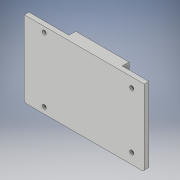
# Autodesk Inventor part: BeagleBoneMountingBracket
Saved by Autodesk Inventor 2019.3 (Build 233278000, 278)
## iProperties
Created: 2019-02-16
Part Number: BeagleBoneMountingBracket
Material: Generic
Document SubType Name: Modeling
Designer: mark
Density: 1 g/cm^3
Appearance: Default
Author: mark
Autodesk Inventor part; units mm, degrees
ref_plane "YZ Plane" through (0, 0, 0) normal (1, 0, 0) x (0, 1, 0)
ref_plane "XZ Plane" through (0, 0, 0) normal (0, 1, 0) x (-1, 0, 0)
ref_plane "XY Plane" through (0, 0, 0) normal (0, 0, 1) x (1, 0, 0)
sketch "Sketch1" plane through (0, 0, 0) normal (0, 0, 1) x (1, 0, 0)
  line L0 (0, 0) -> (90, 0)
  line L1 (90, 0) -> (90, 57)
  line L2 (90, 57) -> (0, 57)
  line L3 (0, 57) -> (0, 0)
  circle A0 centre (15, 53) radius 1.55
  circle A1 centre (15, 4.74) radius 1.55
  circle A2 centre (80.699, 49.825) radius 1.55
  circle A3 centre (80.699, 7.915) radius 1.55
  dimension "d0" = 57
  dimension "d1" = 90
  dimension "d2" = 3.1
  dimension "d3" = 3.1
  dimension "d4" = 3.1
  dimension "d5" = 3.1
  dimension "d6" = 4
  dimension "d7" = 15
  dimension "d8" = 48.26
  dimension "d9" = 15
  dimension "d10" = 80.699
  dimension "d11" = 7.175
  dimension "d12" = 41.91
  dimension "d13" = 80.699
  constraints: 8 end point, 4 centre point, 2 horizontal, 2 vertical
  measures "d0" distance between parallel lines of L0 L2
  measures "d1" distance between parallel lines of L1 L3
  measures "d2" diameter of A0
  measures "d3" diameter of A1
  measures "d4" diameter of A2
  measures "d5" diameter of A3
  measures "d6" distance from line of L2 A0.centre
  measures "d7" distance from line of A0.centre L3
  measures "d8" distance of A1.centre A0.centre
  measures "d9" distance from line of A1.centre L3
  measures "d10" distance from line of L3 A2.centre
  measures "d11" distance from line of L2 A2.centre
  measures "d12" distance of A3.centre A2.centre
  measures "d13" distance from line of A3.centre L3
extrude "Extrusion1" add sketch "Sketch1" along normal blind 3.5
sketch "Sketch2" plane through (0, 0, 0) normal (0, 0, -1) x (-1, 0, 0)
  line L0 (-70, 35) -> (-30, 35)
  line L1 (-30, 35) -> (-30, 57)
  line L2 (-30, 57) -> (-70, 57)
  line L3 (-70, 57) -> (-70, 35)
  line L4 (0, 0) -> (-90, 0) projected
  line L5 (-90, 57) -> (0, 57) projected
  line L6 (-90, 0) -> (-90, 57) projected
  dimension "d16" = 35
  dimension "d17" = 40
  dimension "d18" = 20
  constraints: 8 end point, 2 horizontal, 2 vertical, 1 collinear
  measures "d16" distance between parallel lines of L0 L4
  measures "d17" distance between parallel lines of L1 L3
  measures "d18" distance between parallel lines of L6 L3
extrude "Extrusion2" add sketch "Sketch2" along normal blind 5.1
sketch "Sketch3" plane through (30, 35, 0) normal (0, -1, 0) x (1, 0, 0)
  line L0 (0, -5.1) -> (40, -5.1)
  line L1 (40, -5.1) -> (40, -3.1)
  line L2 (40, -3.1) -> (0, -3.1)
  line L3 (0, -3.1) -> (0, -5.1)
  line L4 (40, -5.1) -> (0, -5.1) projected
  line L5 (0, 0) -> (0, -5.1) projected
  line L6 (40, 0) -> (40, -5.1) projected
  line L7 (-30, 0) -> (60, 0) projected
  dimension "d21" = 3.1
  constraints: 8 end point, 3 collinear
  measures "d21" distance between parallel lines of L7 L2
extrude "Extrusion3" add sketch "Sketch3" along normal blind 25 contours L3 L2 L1 L0
chamfer "Chamfer1" distance 5 angle 45 2 edges at (70, 10, -4.1) (30, 10, -4.1)
chamfer "Chamfer2" distance 1 angle 45 2 edges at (90, 0, 1.75) (0, 0, 1.75)
chamfer "Chamfer3" distance 2 angle 45 4 edges at (13.45, 53, 0) (13.45, 4.74, 0) (79.149, 49.825, 0) (79.149, 7.915, 0)
body "Solid1"
